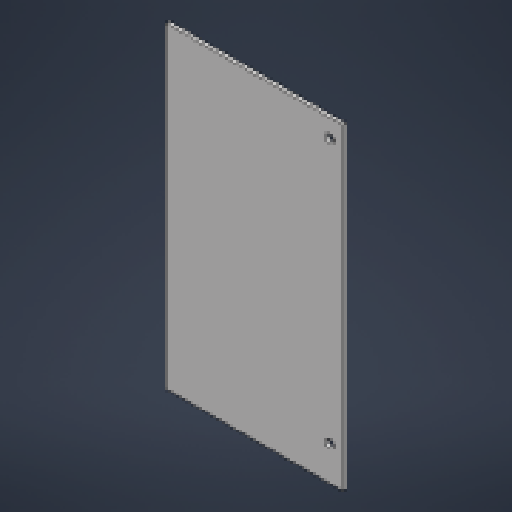
# Autodesk Inventor part: Cata basket polycarb
Saved by Autodesk Inventor 2023.2 (Build 272271030, 271C)
## iProperties
Created: 2023-05-19
Part Number: Cata basket polycarb
Material: Polycarbonate, Clear
Document SubType Name: Modeling
Designer: Main Account
Density: 1.2 g/cm^3
Appearance: Polycarbonate - Clear
Author: Main Account
Autodesk Inventor part; units mm, degrees
ref_plane "YZ Plane" through (0, 0, 0) normal (1, 0, 0) x (0, 1, 0)
ref_plane "XZ Plane" through (0, 0, 0) normal (0, 1, 0) x (-1, 0, 0)
ref_plane "XY Plane" through (0, 0, 0) normal (0, 0, 1) x (1, 0, 0)
sketch "Sketch1" plane through (0, 0, 0) normal (0, 0, 1) x (1, 0, 0)
  line L0 (-50.2524, -73.9518) -> (22.1376, -73.9518)
  line L1 (28.4876, -67.6018) -> (28.4876, 72.0982)
  line L2 (22.1376, 78.4482) -> (-50.2524, 78.4482)
  line L3 (-56.6024, 72.0982) -> (-56.6024, -67.6018)
  line L4 (22.1376, -57.4418) -> (22.1376, 69.5582) construction
  circle A0 centre (22.1376, -57.4418) radius 2.0828
  circle A1 centre (22.1376, 69.5582) radius 2.0828
  arc A2 (22.1376, -73.9518) -> (28.4876, -67.6018) centre (22.1376, -67.6018) ccw
  arc A3 (28.4876, 72.0982) -> (22.1376, 78.4482) centre (22.1376, 72.0982) ccw
  arc A4 (-50.2524, 78.4482) -> (-56.6024, 72.0982) centre (-50.2524, 72.0982) ccw
  arc A5 (-56.6024, -67.6018) -> (-50.2524, -73.9518) centre (-50.2524, -67.6018) ccw
  point P0 (0, 0)
  point P1 (-56.6024, -73.9518)
  point P2 (28.4876, 78.4482)
  point P3 (28.4876, -73.9518)
  point P4 (-56.6024, 78.4482)
  dimension "d0" = 85.09
  dimension "d1" = 152.4
  dimension "d2" = 127
  dimension "d3" = 6.35
  dimension "d4" = 16.51
  dimension "d5" = 4.1656
  dimension "d6" = 4.1656
  dimension "d9" = 6.35
  constraints: 10 end point, 8 point on circle, 8 point on line, 8 tangent, 6 centre point, 3 equal radius, 2 coincident, 2 parallel, 1 horizontal, 1 perpendicular, 1 vertical
  measures "d0" distance of point (-56.602, 78.448) point (28.488, 78.448)
  measures "d1" distance of point (28.488, 78.448) point (28.488, -73.952)
  measures "d2" distance of L4.start L4.end
  measures "d3" distance between parallel lines of L1 L4
  measures "d4" distance from line of L0 L4.start
  measures "d5" diameter of A0
  measures "d6" diameter of A1
  measures "d9" radius of A2
extrude "Extrusion1" add sketch "Sketch1" along normal blind 1.5875
body "Solid1"
